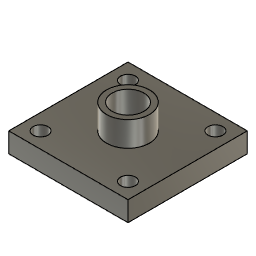
flange_bearing v6 (Autodesk Fusion 360 design; units mm, degrees)
Autodesk Fusion 360 part; units mm, degrees
note: some values were not read from the file. Set by a fixed rule: which sketch regions a step uses.
sketch "Sketch4" plane through (0, 0, 0) normal (0, 0, 1) x (1, 0, 0)
  line L0 (0, 0) -> (95.25, 0)
  line L1 (95.25, 0) -> (95.25, 95.25)
  line L2 (95.25, 95.25) -> (0, 95.25)
  line L3 (0, 95.25) -> (0, 0)
  dimension "d17" = 95.25
  dimension "d18" = 95.25
  constraint horizontal L0
  constraint vertical L1
  constraint horizontal L2
  constraint vertical L3
  constraint coincident L0.start L3.end
  measures "d17" distance of L0.start L0.end
  measures "d18" distance of L0.start L2.end
extrude "Extrude4" add sketch "Sketch4" along normal blind 15.875
sketch "Sketch5" plane through (0, 0, 15.875) normal (0, 0, 1) x (-1, 0, 0)
  line L0 (0, -95.25) -> (0, 0)
  line L1 (0, 0) -> (-95.25, 0)
  line L2 (-95.25, 0) -> (-95.25, -95.25)
  line L3 (-95.25, -95.25) -> (0, -95.25)
  line L4 (0, -95.25) -> (-47.625, -95.25)
  line L5 (-47.625, -95.25) -> (-47.625, -47.625)
  line L6 (-47.625, -47.625) -> (0, -47.625)
  line L7 (0, -47.625) -> (0, -95.25)
  circle A0 centre (-47.625, -47.625) radius 12.7
  dimension "d21" = 47.625
  dimension "d22" = 47.625
  dimension "d23" = 25.4
  constraint horizontal L4
  constraint vertical L5
  constraint horizontal L6
  constraint vertical L7
  constraint coincident L0.start L3.end
  constraint coincident L5.end L6.start
  measures "d21" distance of L0.start L4.end
  measures "d22" distance of L0.start L6.end
  measures "d23" diameter of A0
extrude "Extrude5" cut sketch "Sketch5" against normal blind 25 contours L5 L6 A0 | L5 L6 A0
sketch "Sketch6" plane through (0, 0, 15.875) normal (0, 0, 1) x (-1, 0, 0)
  circle A0 centre (-47.625, -47.625) radius 12.7
  line L0 (0, -95.25) -> (0, 0)
  line L1 (0, 0) -> (-95.25, 0)
  line L2 (-95.25, 0) -> (-95.25, -95.25)
  line L3 (-95.25, -95.25) -> (0, -95.25)
  circle A1 centre (-47.625, -47.625) radius 17.1179
  constraint concentric A0 A1
extrude "Extrude6" add sketch "Sketch6" along normal blind 19.8438 contours A1
sketch "Sketch7" plane through (0, 0, 15.875) normal (0, 0, 1) x (-1, 0, 0)
  circle A0 centre (-47.625, -47.625) radius 17.1179
  line L0 (0, -95.25) -> (0, 0)
  line L1 (0, 0) -> (-95.25, 0)
  line L2 (-95.25, 0) -> (-95.25, -95.25)
  line L3 (-95.25, -95.25) -> (0, -95.25)
  circle A1 centre (-47.625, -47.625) radius 34.925
  line L4 (-47.625, -95.25) -> (-47.625, -82.55)
  line L5 (0, -50) -> (-12.7808, -50)
  line L6 (0, -95.25) -> (-12.7, -95.25)
  line L7 (-12.7, -95.25) -> (-12.7, -82.55)
  line L8 (-12.7, -82.55) -> (0, -82.55)
  line L9 (0, -82.55) -> (0, -95.25)
  line L10 (-95.25, -95.25) -> (-82.55, -95.25)
  line L11 (-82.55, -95.25) -> (-82.55, -82.55)
  line L12 (-82.55, -82.55) -> (-95.25, -82.55)
  line L13 (-95.25, -82.55) -> (-95.25, -95.25)
  line L14 (0, 0) -> (-12.7, 0)
  line L15 (-12.7, 0) -> (-12.7, -12.7)
  line L16 (-12.7, -12.7) -> (0, -12.7)
  line L17 (0, -12.7) -> (0, 0)
  line L18 (-95.25, 0) -> (-82.55, 0)
  line L19 (-82.55, 0) -> (-82.55, -12.7)
  line L20 (-82.55, -12.7) -> (-95.25, -12.7)
  line L21 (-95.25, -12.7) -> (-95.25, 0)
  circle A2 centre (-12.7, -82.55) radius 4.7625
  circle A3 centre (-82.55, -82.55) radius 4.7625
  circle A4 centre (-12.7, -12.7) radius 4.7625
  circle A5 centre (-82.55, -12.7) radius 4.7625
  dimension "d28" = 69.85
  dimension "d29" = 12.7
  dimension "d30" = 12.7
  dimension "d31" = 12.7
  dimension "d32" = 12.7
  dimension "d33" = 12.7
  dimension "d34" = 12.7
  dimension "d35" = 12.7
  dimension "d36" = 12.7
  dimension "d37" = 9.525
  dimension "d38" = 9.525
  dimension "d39" = 9.525
  dimension "d40" = 9.525
  constraint concentric A0 A1
  constraint midpoint L3 L4.start
  constraint coincident A1 L4.end
  constraint perpendicular L3 L4
  constraint coincident L0 L5.start
  constraint coincident A1 L5.end
  constraint perpendicular L0 L5
  constraint horizontal L6
  constraint vertical L7
  constraint horizontal L8
  constraint vertical L9
  constraint coincident L0.start L3.end
  constraint horizontal L10
  constraint vertical L11
  constraint horizontal L12
  constraint vertical L13
  constraint coincident L2.end L3.start
  constraint horizontal L14
  constraint vertical L15
  constraint horizontal L16
  constraint vertical L17
  constraint coincident L0.end L1.start
  constraint horizontal L18
  constraint vertical L19
  constraint horizontal L20
  constraint vertical L21
  constraint coincident L1.end L2.start
  constraint coincident L7.end L8.start
  constraint coincident L11.end L12.start
  constraint coincident L15.end L16.start
  constraint coincident L19.end L20.start
  measures "d28" diameter of A1
  measures "d29" distance of L0.start L6.end
  measures "d30" distance of L0.start L8.end
  measures "d31" distance of L2.end L10.end
  measures "d32" distance of L2.end L12.end
  measures "d33" distance of L0.end L14.end
  measures "d34" distance of L0.end L16.end
  measures "d35" distance of L1.end L18.end
  measures "d36" distance of L1.end L20.end
  measures "d37" diameter of A2
  measures "d38" diameter of A3
  measures "d39" diameter of A4
  measures "d40" diameter of A5
extrude "Extrude7" cut sketch "Sketch7" against normal blind 30 contours L7 L8 A2 | L7 L8 A2 | L15 L16 A4 | L15 L16 A4 | L11 L12 A3 | L11 L12 A3 | L19 L20 A5 | L19 L20 A5
sketch "Sketch8" plane through (0, 0, 15.875) normal (0, 0, 1) x (-1, 0, 0)
  circle A0 centre (-12.7, -12.7) radius 4.7625
  circle A1 centre (-82.55, -12.7) radius 4.7625
  circle A2 centre (-12.7, -82.55) radius 4.7625
  circle A3 centre (-82.55, -82.55) radius 4.7625
  circle A4 centre (-47.625, -47.625) radius 17.1179
  line L0 (0, -95.25) -> (0, 0)
  line L1 (0, 0) -> (-95.25, 0)
  line L2 (-95.25, 0) -> (-95.25, -95.25)
  line L3 (-95.25, -95.25) -> (0, -95.25)
  circle A5 centre (-12.7, -12.7) radius 5.953
  circle A6 centre (-12.7, -82.55) radius 5.953
  circle A7 centre (-82.55, -82.55) radius 5.953
  circle A8 centre (-82.55, -12.7) radius 5.953
  dimension "d43" = 11.906
  dimension "d44" = 11.906
  dimension "d45" = 11.906
  dimension "d46" = 11.906
  constraint concentric A0 A5
  constraint concentric A2 A6
  constraint concentric A3 A7
  constraint concentric A1 A8
  measures "d43" diameter of A5
  measures "d44" diameter of A6
  measures "d45" diameter of A7
  measures "d46" diameter of A8
extrude "Extrude8" cut sketch "Sketch8" against normal blind 35 contours A5 | A6 | A7 | A8
equation "d21 = ( 95.25 / 2 ) * 1 mm"
equation "d22 = ( 95.25 / 2 ) * 1 mm"
equation "d23 = ( 12.7 * 2 ) * 1 mm"
